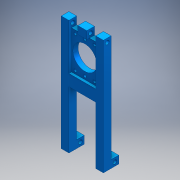
# Autodesk Inventor part: framesideRight
Saved by Autodesk Inventor 2016 (Build 200138000, 138)
## iProperties
Created: 2016-05-18
Part Number: framesideRight
Material: ABS Plastic
Document SubType Name: Modeling
Designer: hesaon
Density: 1.06 g/cm^3
Appearance: Smooth - White
Author: hesaon
Autodesk Inventor part; units mm, degrees
ref_plane "YZ Plane" through (0, 0, 0) normal (1, 0, 0) x (0, 1, 0)
ref_plane "XZ Plane" through (0, 0, 0) normal (0, 1, 0) x (-1, 0, 0)
ref_plane "XY Plane" through (0, 0, 0) normal (0, 0, 1) x (1, 0, 0)
sketch "Sketch1" plane through (0, 0, 0) normal (0, 1, 0) x (-1, 0, 0)
  line L0 (0, 0) -> (66, 0)
  line L1 (66, 0) -> (66, -180)
  line L2 (66, -180) -> (0, -180)
  line L3 (0, -180) -> (0, 0)
  line L4 (54, -12) -> (12, -12)
  line L5 (12, -168) -> (54, -168)
  line L6 (54, -72) -> (12, -72)
  line L7 (54, -90) -> (12, -90)
  line L8 (54, -168) -> (54, -90)
  line L9 (54, -72) -> (54, -12)
  line L10 (12, -12) -> (12, -72)
  line L11 (12, -90) -> (12, -168)
  dimension "d0" = 66
  dimension "d1" = 180
  dimension "d3" = 42
  dimension "d4" = 12
  dimension "d5" = 12
  dimension "d6" = 60
  dimension "d7" = 18
  dimension "d8" = 12
  dimension "d9" = 12
  constraints: 24 end point, 7 perpendicular, 6 parallel, 2 horizontal, 1 collinear
  measures "d0" distance of L1.end L2.end
  measures "d1" distance of L0.end L1.end
  measures "d3" distance of L5.start L5.end
  measures "d4" distance from line of L2 L5.start
  measures "d5" distance from line of L1 L5.end
  measures "d6" distance of L4.end L6.end
  measures "d7" distance of L7.end L6.end
  measures "d8" distance between parallel lines of L0 L4
  measures "d9" distance from line of L3 L4.end
extrude "Extrusion1" add sketch "Sketch1" along normal blind 12
sketch "Sketch2" plane through (0, 12, 0) normal (0, 1, 0) x (1, 0, 0)
  circle A0 centre (-48, 17) radius 2.1
  circle A1 centre (-33, 17) radius 2.1
  circle A2 centre (-18, 17) radius 2.1
  circle A3 centre (-48, 67) radius 2.1
  circle A4 centre (-33, 67) radius 2.1
  circle A5 centre (-18, 67) radius 2.1
  line L0 (-12, 12) -> (-12, 72) projected
  line L1 (-12, 12) -> (-54, 12) projected
  line L2 (-12, 72) -> (-54, 72) projected
  line L3 (-54, 12) -> (-12, 12) projected
  line L4 (-54, 12) -> (-54, 72)
  line L5 (-54, 12) -> (-54, 72) projected
  line L6 (-54, 12) -> (-12, 12)
  line L7 (-12, 72) -> (-12, 12) projected
  line L8 (-12, 12) -> (-12, 72)
  line L9 (-12, 72) -> (-54, 72)
  dimension "d12" = 4.2
  dimension "d13" = 4.2
  dimension "d15" = 4.2
  dimension "d16" = 4.2
  dimension "d17" = 4.2
  dimension "d42" = 21
  dimension "d43" = 21
  dimension "d44" = 15
  dimension "d45" = 15
  dimension "d46" = 15
  dimension "d47" = 15
  dimension "d48" = 4.2
  dimension "d49" = 5
  dimension "d50" = 5
  dimension "d51" = 5
  dimension "d52" = 5
  dimension "d53" = 5
  constraints: 8 end point, 6 centre point, 2 perpendicular, 1 collinear, 1 vertical
  measures "d12" diameter of A0
  measures "d13" diameter of A1
  measures "d15" diameter of A3
  measures "d16" diameter of A4
  measures "d17" diameter of A5
  measures "d42" distance from line of L0 A1.centre
  measures "d43" distance from line of L0 A4.centre
  measures "d44" distance of A4.centre A5.centre
  measures "d45" distance of A4.centre A3.centre
  measures "d46" distance of A1.centre A0.centre
  measures "d47" distance of A2.centre A1.centre
  measures "d48" diameter of A2
  measures "d49" distance from line of L1 A1.centre
  measures "d50" distance from line of L2 A4.centre
  measures "d51" distance from line of L2 A5.centre
  measures "d52" distance from line of L2 A3.centre
  measures "d53" distance from line of L1 A0.centre
extrude "Extrusion2" add sketch "Sketch2" against normal blind 8
sketch "Sketch3" plane through (0, 4, 0) normal (0, -1, 0) x (1, 0, 0)
  circle A0 centre (-33, -42) radius 18.75
  line L0 (-12, -12) -> (-12, -72) projected
  line L1 (-12, -72) -> (-54, -72) projected
  point P0 (0, 0)
  dimension "d56" = 37.5
  dimension "d57" = 21
  dimension "d58" = 30
  constraints: 1 centre point
  measures "d56" diameter of A0
  measures "d57" distance from line of L0 A0.centre
  measures "d58" distance from line of L1 A0.centre
extrude "Extrusion3" cut sketch "Sketch3" against normal up to next
sketch "Sketch4" plane through (0, 0, 0) normal (0, -1, 0) x (1, 0, 0)
  line L0 (-66, 0) -> (-66, -180) projected
  line L1 (-26, 0) -> (-12, 0)
  line L2 (-12, 0) -> (-12, -12)
  line L3 (-12, -12) -> (-26, -12)
  line L4 (-26, -12) -> (-26, 0)
  line L5 (-54, 0) -> (-40, 0)
  line L6 (-40, 0) -> (-40, -12)
  line L7 (-40, -12) -> (-54, -12)
  line L8 (-54, -12) -> (-54, 0)
  point P0 (-54, -12)
  point P1 (-12, -12)
  dimension "d87" = 14
  dimension "d88" = 12
  dimension "d89" = 14
  dimension "d90" = 12
  constraints: 16 end point, 4 parallel, 2 coincident, 2 horizontal, 2 perpendicular
  measures "d87" distance of L2.end L3.end
  measures "d88" distance of L1.end L2.end
  measures "d89" distance of L6.end L7.end
  measures "d90" distance of L5.end L6.end
extrude "Extrusion5" cut sketch "Sketch4" against normal up to next
sketch "Sketch5" plane through (0, 0, 0) normal (1, 0, 0) x (0, 0, -1)
  line L0 (0, 0) -> (12, 0)
  line L1 (12, 0) -> (12, 12)
  line L2 (12, 12) -> (0, 12)
  line L3 (0, 12) -> (0, 0)
  circle A0 centre (6, 6) radius 3
  dimension "d93" = 12
  dimension "d94" = 12
  dimension "d95" = 6
  dimension "d96" = 6
  dimension "d97" = 6
  constraints: 8 end point, 2 parallel, 1 centre point, 1 coincident, 1 horizontal, 1 perpendicular
  measures "d93" distance of L2.end L1.end
  measures "d94" distance of L1.end L0.end
  measures "d95" diameter of A0
  measures "d96" distance from line of L2 A0.centre
  measures "d97" distance from line of L3 A0.centre
extrude "Extrusion6" cut sketch "Sketch5" against normal blind 66 contours A0
sketch "Sketch6" plane through (0, 0, 0) normal (0, -1, 0) x (1, 0, 0)
  line L0 (-54, -90) -> (-54, -168) projected
  line L1 (-54, -168) -> (-12, -168)
  line L2 (-12, -168) -> (-12, -180)
  line L3 (-12, -180) -> (-54, -180)
  line L4 (-54, -180) -> (-54, -168)
  point P0 (0, 0)
  dimension "d100" = 42
  dimension "d101" = 12
  constraints: 8 end point, 2 parallel, 1 horizontal, 1 perpendicular
  measures "d100" distance of L2.end L3.end
  measures "d101" distance of L1.end L2.end
extrude "Extrusion7" cut sketch "Sketch6" against normal up to next
sketch "Sketch13" plane through (0, 12, 0) normal (0, 1, 0) x (1, 0, 0)
  line L0 (0, 180) -> (-12, 180) projected
  line L1 (0, 180) -> (-12, 180)
  line L2 (-12, 180) -> (-12, 168)
  line L3 (-12, 168) -> (0, 168)
  line L4 (0, 168) -> (0, 180)
  line L5 (-66, 180) -> (-54, 180) projected
  line L6 (-54, 180) -> (-66, 180)
  line L7 (-66, 180) -> (-66, 168)
  line L8 (-66, 168) -> (-54, 168)
  line L9 (-54, 168) -> (-54, 180)
  point P0 (0, 0)
  dimension "d136" = 12
  dimension "d137" = 12
  dimension "d138" = 12
  dimension "d139" = 12
  constraints: 16 end point, 4 parallel, 2 horizontal, 2 perpendicular
  measures "d136" distance of L3.end L2.end
  measures "d137" distance of L2.end L1.end
  measures "d138" distance of L8.end L7.end
  measures "d139" distance of L7.end L6.end
extrude "Extrusion13" add sketch "Sketch13" along normal blind 12
sketch "Sketch14" plane through (0, 0, 0) normal (1, 0, 0) x (0, 0, -1)
  circle A0 centre (174, 18) radius 3
  line L0 (168, 12) -> (168, 24) projected
  line L1 (168, 24) -> (180, 24) projected
  point P0 (0, 0)
  dimension "d142" = 6
  dimension "d143" = 6
  dimension "d144" = 6
  constraints: 1 centre point
  measures "d142" diameter of A0
  measures "d143" distance from line of L0 A0.centre
  measures "d144" distance from line of L1 A0.centre
extrude "Extrusion14" cut sketch "Sketch14" against normal blind 66
sketch "Sketch15" plane through (-12, 0, -90) normal (0, 0, -1) x (-1, 0, 0)
  circle A0 centre (7, 6) radius 3
  circle A1 centre (24, 6) radius 3
  line L0 (0, 0) -> (0, 24) projected
  line L1 (0, 12) -> (42, 12) projected
  point P0 (-12, 0)
  dimension "d147" = 6
  dimension "d148" = 6
  dimension "d149" = 7
  dimension "d150" = 17
  dimension "d151" = 6
  dimension "d152" = 6
  constraints: 2 centre point
  measures "d147" diameter of A0
  measures "d148" diameter of A1
  measures "d149" distance from line of L0 A0.centre
  measures "d150" distance of A1.centre A0.centre
  measures "d151" distance from line of L1 A0.centre
  measures "d152" distance from line of L1 A1.centre
extrude "Extrusion15" cut sketch "Sketch15" against normal blind 6
body "Solid1"
